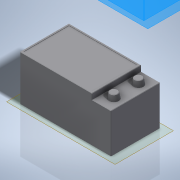
# Autodesk Inventor part: Bateria de camion
Saved by Autodesk Inventor 2022 (Build 260153000, 153)
## iProperties
Created: 2021-09-12
Part Number: Bateria de camion
Material: Generic
Document SubType Name: Modeling
Designer: ARMU
Density: 1 g/cm^3
Appearance: Default
Author: ARMU
Autodesk Inventor part; units mm, degrees
ref_plane "YZ Plane" through (0, 0, 0) normal (1, 0, 0) x (0, 1, 0)
ref_plane "XZ Plane" through (0, 0, 0) normal (0, 1, 0) x (-1, 0, 0)
ref_plane "XY Plane" through (0, 0, 0) normal (0, 0, 1) x (1, 0, 0)
sketch "Sketch6" plane through (0, 0, 0) normal (0, 1, 0) x (-1, 0, 0)
  line L0 (227, 0) -> (0, 0)
  line L1 (0, 0) -> (0, -314)
  line L2 (0, -314) -> (227, -314)
  line L3 (227, -314) -> (227, 0)
  dimension "d30" = 227
  dimension "d31" = 314
  constraints: 8 end point, 2 parallel, 1 coincident, 1 horizontal, 1 perpendicular
  measures "d30" distance of L2.end L1.end
  measures "d31" distance of L1.end L0.end
extrude "Extrusion5" add sketch "Sketch6" along normal blind 417
sketch "Sketch7" plane through (0, 0, 0) normal (0, -1, 0) x (1, 0, 0)
  line L0 (-217, -20) -> (-10, -20)
  line L1 (-10, -20) -> (-10, -294)
  line L2 (-10, -294) -> (-217, -294)
  line L3 (-217, -294) -> (-217, -20)
  line L4 (-227, -314) -> (-227, 0) projected
  line L5 (0, 0) -> (0, -314) projected
  line L6 (0, -314) -> (-227, -314) projected
  line L7 (-227, 0) -> (0, 0) projected
  dimension "d34" = 10
  dimension "d35" = 10
  dimension "d36" = 20
  dimension "d37" = 20
  constraints: 8 end point, 2 parallel, 1 horizontal, 1 perpendicular
  measures "d34" distance between parallel lines of L3 L4
  measures "d35" distance between parallel lines of L5 L1
  measures "d36" distance between parallel lines of L6 L2
  measures "d37" distance between parallel lines of L7 L0
extrude "Extrusion6" cut sketch "Sketch7" against normal blind 10 contours L0 L1 L2 L3
sketch "Sketch8" plane through (0, 417, 0) normal (0, 1, 0) x (1, 0, 0)
  line L0 (-217, 20) -> (-10, 20)
  line L1 (-10, 20) -> (-10, 294)
  line L2 (-10, 294) -> (-217, 294)
  line L3 (-217, 294) -> (-217, 20)
  line L4 (0, 314) -> (-227, 314) projected
  line L5 (-227, 0) -> (0, 0) projected
  line L6 (0, 0) -> (0, 314) projected
  line L7 (-227, 314) -> (-227, 0) projected
  dimension "d40" = 20
  dimension "d41" = 20
  dimension "d42" = 10
  dimension "d43" = 10
  constraints: 8 end point, 2 parallel, 1 horizontal, 1 perpendicular
  measures "d40" distance between parallel lines of L4 L2
  measures "d41" distance between parallel lines of L5 L0
  measures "d42" distance between parallel lines of L6 L1
  measures "d43" distance between parallel lines of L7 L3
extrude "Extrusion7" cut sketch "Sketch8" against normal blind 10 contours L3 L2 L1 L0
sketch "Sketch9" plane through (-227, 0, 0) normal (0, 0, 1) x (1, 0, 0)
  line L0 (0, 392.5) -> (227, 392.5)
  line L1 (227, 392.5) -> (227, 24.5)
  line L2 (227, 24.5) -> (0, 24.5)
  line L3 (0, 24.5) -> (0, 392.5)
  line L4 (0, 417) -> (227, 417) projected
  line L5 (0, 0) -> (227, 0) projected
  line L6 (0, 0) -> (0, 417) projected
  line L7 (227, 0) -> (227, 417) projected
  dimension "d46" = 24.5
  dimension "d47" = 24.5
  dimension "d48" = 0
  dimension "d49" = 0
  constraints: 8 end point, 2 parallel, 1 horizontal, 1 perpendicular
  measures "d46" distance between parallel lines of L4 L0
  measures "d47" distance between parallel lines of L5 L2
  measures "d48" distance between parallel lines of L3 L6
  measures "d49" distance between parallel lines of L7 L1
extrude "Extrusion8" cut sketch "Sketch9" against normal blind 5 contours L0 L1 L2 L3
sketch "Sketch10" plane through (0, 0, 0) normal (1, 0, 0) x (0, 0, -1)
  line L0 (29.5, 24.5) -> (314, 24.5)
  line L1 (314, 24.5) -> (314, 392.5)
  line L2 (314, 392.5) -> (29.5, 392.5)
  line L3 (29.5, 392.5) -> (29.5, 24.5)
  line L4 (5, 24.5) -> (0, 24.5) projected
  line L5 (0, 392.5) -> (5, 392.5) projected
  line L6 (5, 392.5) -> (5, 24.5) projected
  line L7 (314, 0) -> (314, 417) projected
  point P0 (0, 0)
  dimension "d52" = 0
  dimension "d53" = 0
  dimension "d54" = 24.5
  dimension "d55" = 0
  constraints: 8 end point, 2 parallel, 1 horizontal, 1 perpendicular
  measures "d52" distance between parallel lines of L4 L0
  measures "d53" distance between parallel lines of L5 L2
  measures "d54" distance between parallel lines of L6 L3
  measures "d55" distance between parallel lines of L1 L7
extrude "Extrusion9" cut sketch "Sketch10" against normal blind 2
sketch "Sketch11" plane through (-227, 0, -314) normal (-1, 0, 0) x (0, 0, 1)
  line L0 (284.5, 24.5) -> (284.5, 392.5) projected
  line L1 (0, 392.5) -> (0, 24.5) projected
  line L2 (284.5, 392.5) -> (0, 392.5)
  line L3 (0, 392.5) -> (0, 24.5)
  line L4 (0, 24.5) -> (284.5, 24.5)
  line L5 (284.5, 24.5) -> (284.5, 392.5)
  point P0 (314, 0)
  constraints: 8 end point, 2 parallel, 1 horizontal, 1 perpendicular
extrude "Extrusion10" cut sketch "Sketch11" against normal blind 2
sketch "Sketch12" plane through (0, 0, -314) normal (0, 0, -1) x (-1, 0, 0)
  line L0 (225, 392.5) -> (227, 392.5) projected
  line L1 (2, 24.5) -> (0, 24.5) projected
  line L2 (225, 392.5) -> (2, 392.5)
  line L3 (2, 392.5) -> (2, 24.5)
  line L4 (2, 24.5) -> (225, 24.5)
  line L5 (225, 24.5) -> (225, 392.5)
  point P0 (0, 0)
  constraints: 8 end point, 2 parallel, 1 horizontal, 1 perpendicular
extrude "Extrusion11" cut sketch "Sketch12" against normal blind 2
sketch "Sketch13" plane through (-227, 0, -5) normal (0, 0, 1) x (1, 0, 0)
  line L0 (88.5, 64.5) -> (138.5, 64.5)
  line L1 (138.5, 64.5) -> (138.5, 114.5)
  line L2 (138.5, 114.5) -> (88.5, 114.5)
  line L3 (88.5, 114.5) -> (88.5, 64.5)
  line L4 (40, 327.5) -> (90, 327.5)
  line L5 (90, 327.5) -> (90, 377.5)
  line L6 (90, 377.5) -> (40, 377.5)
  line L7 (40, 377.5) -> (40, 327.5)
  line L8 (137, 327.5) -> (187, 327.5)
  line L9 (187, 327.5) -> (187, 377.5)
  line L10 (187, 377.5) -> (137, 377.5)
  line L11 (137, 377.5) -> (137, 327.5)
  line L12 (227, 392.5) -> (227, 24.5) projected
  line L13 (0, 24.5) -> (0, 392.5) projected
  line L14 (88.5, 114.5) -> (138.5, 64.5) construction
  line L15 (88.5, 64.5) -> (138.5, 114.5) construction
  line L16 (90, 377.5) -> (137, 327.5) construction
  line L17 (90, 327.5) -> (137, 377.5) construction
  line L18 (113.5, 352.5) -> (113.5, -96.0113) construction
  line L19 (113.5, 352.5) -> (562.0113, 352.5) construction
  line L20 (227, 24.5) -> (0, 24.5) construction
  line L21 (0, 392.5) -> (227, 392.5) construction
  point P0 (227, 0)
  point P1 (113.5, 89.5)
  dimension "d62" = 50
  dimension "d63" = 50
  dimension "d64" = 50
  dimension "d65" = 227
  dimension "d66" = 40
  dimension "d67" = 40
  dimension "d68" = 90
  dimension "d69" = 40
  dimension "d70" = 50
  dimension "d71" = 50
  dimension "d72" = 40
  constraints: 36 end point, 6 parallel, 4 horizontal, 4 perpendicular, 2 midpoint, 2 point on line, 1 collinear
  measures "d62" distance of L6.end L4.start
  measures "d63" distance of L5.end L6.end
  measures "d64" distance of L9.end L10.end
  measures "d65" distance between parallel lines of L12 L13
  measures "d66" distance between parallel lines of L7 L13
  measures "d67" distance between parallel lines of L12 L9
  measures "d68" angle of L18 L19
  measures "d69" distance between parallel lines of L0 L20
  measures "d70" distance of L2.end L0.start
  measures "d71" distance of L1.end L2.end
  measures "d72" distance from line of L21 L18.start
extrude "Extrusion12" add sketch "Sketch13" along normal blind 1
sketch "Sketch14" plane through (-227, 0, -4) normal (0, 0, 1) x (1, 0, 0)
  circle A0 centre (106.4289, 82.4289) radius 5
  line L0 (40, 327.5) -> (90, 327.5) construction
  line L1 (90, 377.5) -> (90, 327.5) construction
  line L2 (88.5, 64.5) -> (88.5, 114.5) construction
  line L3 (138.5, 64.5) -> (138.5, 114.5) construction
  line L4 (88.5, 64.5) -> (138.5, 114.5) construction
  line L5 (88.5, 114.5) -> (138.5, 114.5) construction
  line L6 (88.5, 114.5) -> (138.5, 64.5) construction
  circle A1 centre (113.5, 89.5) radius 10 construction
  circle A2 centre (120.5711, 96.5711) radius 5
  circle A3 centre (57.9289, 345.4289) radius 5
  line L7 (40, 327.5) -> (90, 377.5) construction
  line L8 (40, 377.5) -> (90, 327.5) construction
  circle A4 centre (65, 352.5) radius 10 construction
  circle A5 centre (72.0711, 359.5711) radius 5
  line L9 (137, 327.5) -> (137, 377.5) projected
  line L10 (137, 327.5) -> (137, 377.5)
  circle A6 centre (154.9289, 345.4289) radius 5
  line L11 (137, 327.5) -> (187, 377.5) construction
  line L12 (137, 377.5) -> (187, 327.5) construction
  circle A7 centre (162, 352.5) radius 10 construction
  circle A8 centre (169.0711, 359.5711) radius 5
  point P0 (227, 0)
  dimension "d75" = 10
  dimension "d79" = 20
  dimension "d80" = 10
  dimension "d84" = 10
  dimension "d85" = 20
  dimension "d86" = 10
  dimension "d87" = 10
  dimension "d88" = 20
  dimension "d89" = 10
  constraints: 14 end point, 9 centre point, 6 point on circle, 6 point on line, 3 midpoint, 1 collinear
  measures "d75" diameter of A0
  measures "d79" diameter of A1
  measures "d80" diameter of A2
  measures "d84" diameter of A3
  measures "d85" diameter of A4
  measures "d86" diameter of A5
  measures "d87" diameter of A6
  measures "d88" diameter of A7
  measures "d89" diameter of A8
extrude "Extrusion13" add sketch "Sketch14" along normal blind 3
fillet "Fillet1" radius 2 9 edges at (-227, 0, -157) (-113.5, 0, -314) (-227, 12.25, -314) (0, 0, -157) (-10, 0, -157) (-113.5, 0, -294) (-217, 0, -157) (-113.5, 0, -20) (-113.5, 0, 0)
fillet "Fillet2" radius 2 7 edges at (-113.5, 417, 0) (-227, 417, -157) (-113.5, 417, -294) (-10, 417, -157) (0, 417, -157) (-113.5, 417, -314) (-113.5, 417, -20)
fillet "Fillet3" radius 2 7 edges at (-113.5, 392.5, 0) (0, 392.5, -2.5) (-227, 392.5, -2.5) (-226.4142, 416.4142, -0.5858) (-227, 403.75, 0) (-0.5858, 416.4142, -0.5858) (0, 403.75, 0)
fillet "Fillet4" radius 2 7 edges at (-113.5, 24.5, 0) (-227, 24.5, -2.5) (-226.4142, 0.5858, -0.5858) (-227, 13.25, 0) (-0.5858, 0.5858, -0.5858) (0, 13.25, 0) (0, 24.5, -2.5)
body "Solid2"
